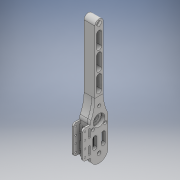
# Autodesk Inventor part: Arm - forearm v2
Saved by Autodesk Inventor 2017 (Build 210142000, 142)
## iProperties
Created: 2016-08-12
Part Number: Arm - forearm v2
Material: Generic
Document SubType Name: Modeling
Designer: Ali
Density: 1 g/cm^3
Appearance: Default
Author: Ali
Autodesk Inventor part; units mm, degrees
ref_plane "YZ Plane" through (0, 0, 0) normal (1, 0, 0) x (0, 1, 0)
ref_plane "XZ Plane" through (0, 0, 0) normal (0, 1, 0) x (-1, 0, 0)
ref_plane "XY Plane" through (0, 0, 0) normal (0, 0, 1) x (1, 0, 0)
sketch "Sketch1" plane through (0, 0, 0) normal (1, 0, 0) x (0, 1, 0)
  line L0 (0, 160) -> (0, -54.4) construction
  line L1 (-8, 160) -> (-8, 40)
  arc A0 (8, 160) -> (-8, 160) centre (0, 160) ccw
  circle A1 centre (0, 0) radius 11
  circle A2 centre (0, 0) radius 17 construction
  arc A3 (8, 40) -> (15.3617, 7.2814) centre (84.3889, 40) ccw
  arc A4 (-15.3617, 7.2814) -> (-8, 40) centre (-84.3889, 40) ccw
  line L2 (0, 0) -> (0, -54.4) construction
  line L3 (-17, 0) -> (-17, -54.4)
  line L4 (17, -54.4) -> (17, 0)
  arc A5 (-17, -54.4) -> (17, -54.4) centre (0, -54.4) ccw
  arc A6 (17, 0) -> (15.3617, 7.2814) centre (0, 0) ccw
  arc A7 (-15.3617, 7.2814) -> (-17, 0) centre (0, 0) ccw
  line L5 (8, 40) -> (8, 160)
  line L6 (-8, 40) -> (8, 40) construction
  point P0 (0, 52.8)
  point P1 (0, -27.2)
  dimension "d0" = 160
  dimension "d1" = 54.4
  dimension "d2" = 22
  dimension "d3" = 6
  dimension "d5" = 34
  dimension "d6" = 16
  dimension "d7" = 40
  constraints: 18 end point, 14 point on circle, 8 centre point, 8 tangent, 3 coincident, 3 vertical, 2 midpoint, 2 parallel, 1 collinear, 1 horizontal, 1 point on line
  measures "d0" distance of point (0, 0) L0.start
  measures "d1" distance of L0.end point (0, 0)
  measures "d2" diameter of A1
  measures "d3" radial gap between concentric circles of A1 A2
  measures "d5" distance between parallel lines of L4 L3
  measures "d6" distance between parallel lines of L5 L1
  measures "d7" distance from line of point (0, 0) L6
extrude "Extrusion1" add sketch "Sketch1" along normal mid plane 20.6
hole "Hole1" at (10.3, 0, 160) direction (-1, 0, 0) diameter 4.3 end through all
sketch "Sketch2" plane through (0, 0, 0) normal (1, 0, 0) x (0, 1, 0)
  circle A0 centre (0, 0) radius 11 projected
extrude "Extrusion2" add sketch "Sketch2" along normal mid plane 6.6
hole "Hole3" at (3.3, 0, 0) direction (-1, 0, 0) diameter 12 end through all
sketch "Sketch3" plane through (10.3, 0, 0) normal (1, 0, 0) x (0, 0, -1)
  line L0 (54.4, 17) -> (0, 17) projected
  arc A0 (54.4, -17) -> (54.4, 17) centre (54.4, 0) ccw projected
  line L1 (0, -17) -> (54.4, -17) projected
  circle A1 centre (0, 0) radius 11 projected
  arc A2 (-7.2814, -15.3617) -> (-40, -8) centre (-40, -84.3889) ccw projected
  arc A3 (-40, 8) -> (-7.2814, 15.3617) centre (-40, 84.3889) ccw projected
  line L2 (-40, 8) -> (-40, -8)
  arc A4 (0, 17) -> (-7.2814, 15.3617) centre (0, 0) ccw projected
  arc A5 (-7.2814, -15.3617) -> (0, -17) centre (0, 0) ccw projected
  constraints: 4 end point, 2 point on circle
extrude "Extrusion3" add sketch "Sketch3" against normal blind 6 separate body
extrude "Extrusion4" cut sketch "Sketch3" against normal blind 6 bodies 1
hole "Hole4" at (10.3, 0, -54.4) direction (-1, 0, 0) diameter 4.3 end through all counterbore diameter 7.1 counterbore depth 4.1 bodies 2 1
sketch "Sketch4" plane through (4.3, 0, 0) normal (1, 0, 0) x (0, 0, -1)
  circle A0 centre (0, 0) radius 11 projected
  line L0 (0, 17) -> (54.4, 17) projected
  arc A1 (54.4, -17) -> (54.4, 17) centre (54.4, 0) ccw projected
  line L1 (54.4, -17) -> (0, -17) projected
  arc A2 (12.3288, -17) -> (12.3288, 17) centre (0, 0) ccw
  dimension "d53" = 10
  constraints: 2 point on circle, 2 point on line, 1 centre point, 1 coincident
  measures "d53" radial gap between concentric circles of A2 A0
extrude "Extrusion5" cut sketch "Sketch4" against normal blind 8.6 contours L0 A1 L1 A2 bodies 1
sketch "Sketch5" plane through (10.3, 0, 0) normal (1, 0, 0) x (0, 0, -1)
  point P0 (0, 0)
  point P1 (-24, 0)
  point P2 (10, 12)
  point P3 (10, -12)
  dimension "d56" = 12
  dimension "d57" = 12
  dimension "d58" = 24
  dimension "d59" = 10
  dimension "d60" = 10
  measures "d56" vertical distance of point (10, 12) point (0, 0)
  measures "d57" vertical distance of point (10, -12) point (0, 0)
  measures "d58" distance of point (0, 0) point (-24, 0)
  measures "d59" horizontal distance of point (10, 12) point (0, 0)
  measures "d60" horizontal distance of point (10, -12) point (0, 0)
hole "Hole5" at (10.3, 0, 0) at (10.3, 0, 24) at (10.3, 12, -10) at (10.3, -12, -10) direction (-1, 0, 0) diameter 3.2 end through all counterbore diameter 6 counterbore depth 3.2 bodies 2 1
sketch "Sketch6" plane through (-10.3, 0, 0) normal (-1, 0, 0) x (0, 0, 1)
  circle A0 centre (-10, 12) radius 1.6 projected
  circle A1 centre (-10, 12) radius 3 projected
  line L0 (-7, 10.2679) -> (-10, 8.5359)
  line L1 (-10, 8.5359) -> (-13, 10.2679)
  line L2 (-13, 10.2679) -> (-13, 13.7321)
  line L3 (-13, 13.7321) -> (-10, 15.4641)
  line L4 (-10, 15.4641) -> (-7, 13.7321)
  line L5 (-7, 13.7321) -> (-7, 10.2679)
  circle A2 centre (-10, -12) radius 1.6 projected
  circle A3 centre (-10, -12) radius 3 projected
  line L6 (-7, -13.7321) -> (-10, -15.4641)
  line L7 (-10, -15.4641) -> (-13, -13.7321)
  line L8 (-13, -13.7321) -> (-13, -10.2679)
  line L9 (-13, -10.2679) -> (-10, -8.5359)
  line L10 (-10, -8.5359) -> (-7, -10.2679)
  line L11 (-7, -10.2679) -> (-7, -13.7321)
  circle A4 centre (24, 0) radius 3 projected
  line L12 (27, -1.7321) -> (24, -3.4641)
  line L13 (24, -3.4641) -> (21, -1.7321)
  line L14 (21, -1.7321) -> (21, 1.7321)
  line L15 (21, 1.7321) -> (24, 3.4641)
  line L16 (24, 3.4641) -> (27, 1.7321)
  line L17 (27, 1.7321) -> (27, -1.7321)
  point P0 (0, 0)
  point P1 (-7, 12)
  point P2 (-7, -12)
  point P3 (27, 0)
  constraints: 36 end point, 3 coincident, 3 horizontal alignment, 3 midpoint, 1 point on line, 42 other
extrude "Extrusion6" cut sketch "Sketch6" against normal blind 5 bodies 1
sketch "Sketch7" plane through (-10.3, 0, 0) normal (-1, 0, 0) x (0, 0, 1)
  circle A0 centre (-54.4, 0) radius 2.15 projected
  circle A1 centre (-54.4, 0) radius 3.55 projected
  line L0 (-50.85, -2.0496) -> (-54.4, -4.0992)
  line L1 (-54.4, -4.0992) -> (-57.95, -2.0496)
  line L2 (-57.95, -2.0496) -> (-57.95, 2.0496)
  line L3 (-57.95, 2.0496) -> (-54.4, 4.0992)
  line L4 (-54.4, 4.0992) -> (-50.85, 2.0496)
  line L5 (-50.85, 2.0496) -> (-50.85, -2.0496)
  point P0 (0, 0)
  point P1 (-50.85, 0)
  constraints: 12 end point, 1 coincident, 1 horizontal alignment, 1 midpoint, 14 other
extrude "Extrusion7" cut sketch "Sketch7" against normal blind 4 bodies 1
sketch "Sketch8" plane through (10.3, 0, 0) normal (1, 0, 0) x (0, 0, -1)
  line L0 (-160, -5.6569) -> (-154.3431, 0)
  line L1 (-154.3431, 0) -> (-160, 5.6569)
  line L2 (-160, 5.6569) -> (-165.6569, 0)
  line L3 (-165.6569, 0) -> (-160, -5.6569)
  line L4 (-154.3431, 0) -> (-165.6569, 0) construction
  circle A0 centre (-160, 0) radius 2.15 projected
  point P0 (0, 0)
  point P1 (-160, 0)
  dimension "d74" = 8
  constraints: 10 end point, 2 parallel, 2 perpendicular, 1 coincident, 1 horizontal, 1 midpoint
  measures "d74" distance between parallel lines of L2 L0
extrude "Extrusion8" cut sketch "Sketch8" against normal blind 4 bodies 1
mirror "Mirror1" about plane through (0, 0, 0) normal (1, 0, 0) of "Extrusion8" bodies 1
sketch "Sketch9" plane through (-10.3, 0, 0) normal (-1, 0, 0) x (0, 0, 1)
  line L0 (-54.4, -17) -> (0, -17) projected
  line L1 (0, 17) -> (-54.4, 17) projected
  line L2 (-25.7926, -8) -> (-41.7926, -8) construction
  line L3 (-25.7926, -4) -> (-41.7926, -4)
  line L4 (-41.7926, -12) -> (-25.7926, -12)
  arc A0 (-25.7926, -12) -> (-25.7926, -4) centre (-25.7926, -8) ccw
  arc A1 (-41.7926, -4) -> (-41.7926, -12) centre (-41.7926, -8) ccw
  line L5 (0, 0) -> (-49.4769, 0)
  line L6 (-25.7926, 8) -> (-41.7926, 8) construction
  line L7 (-25.7926, 4) -> (-41.7926, 4)
  line L8 (-41.7926, 12) -> (-25.7926, 12)
  arc A2 (-25.7926, 4) -> (-25.7926, 12) centre (-25.7926, 8) ccw
  arc A3 (-41.7926, 12) -> (-41.7926, 4) centre (-41.7926, 8) ccw
  point P0 (-33.7926, -8)
  point P1 (-33.7926, 8)
  dimension "d77" = 8
  dimension "d78" = 16
  dimension "d79" = 8
  constraints: 18 end point, 8 point on circle, 7 symmetric about line, 4 centre point, 4 tangent, 2 horizontal, 1 midpoint, 1 parallel, 2 other
  measures "d77" diameter of A1
  measures "d78" distance of L2.start L2.end
  measures "d79" distance between parallel lines of L3 L7
extrude "Extrusion9" cut sketch "Sketch9" against normal through all bodies 1 2
sketch "Sketch10" plane through (-10.3, 0, 0) normal (-1, 0, 0) x (0, 0, 1)
  line L0 (-54.4, -17) -> (0, -17) projected
  line L1 (0, -17) -> (-54.4, -17)
  line L2 (-54.4, -17) -> (-54.4, -31)
  line L3 (-54.4, -31) -> (0, -31)
  line L4 (0, -31) -> (0, -17)
  line L5 (-6, -18.5) -> (-20.1333, -18.5) construction
  line L6 (-6, -17) -> (-20.1333, -17)
  line L7 (-20.1333, -20) -> (-6, -20)
  arc A0 (-6, -20) -> (-6, -17) centre (-6, -18.5) ccw
  arc A1 (-20.1333, -17) -> (-20.1333, -20) centre (-20.1333, -18.5) ccw
  line L8 (-34.2667, -18.5) -> (-48.4, -18.5) construction
  line L9 (-34.2667, -17) -> (-48.4, -17)
  line L10 (-48.4, -20) -> (-34.2667, -20)
  arc A2 (-34.2667, -20) -> (-34.2667, -17) centre (-34.2667, -18.5) ccw
  arc A3 (-48.4, -17) -> (-48.4, -20) centre (-48.4, -18.5) ccw
  point P0 (0, 0)
  point P1 (-13.0667, -18.5)
  point P2 (-41.3333, -18.5)
  dimension "d82" = 14
  dimension "d83" = 3
  dimension "d84" = 1.5
  dimension "d85" = 6
  dimension "d86" = 6
  dimension "d88" = 42.4
  dimension "d89" = 14.1333
  dimension "d90" = 14.1333
  constraints: 24 end point, 8 point on circle, 8 tangent, 4 centre point, 4 parallel, 3 point on line, 2 horizontal, 2 midpoint, 1 collinear, 1 perpendicular
  measures "d82" distance between parallel lines of L3 L0
  measures "d83" diameter of A1
  measures "d84" radius of A2
  measures "d85" distance from line of L4 L5.start
  measures "d86" distance from line of L2 L8.end
  measures "d88" distance of L8.end L5.start
  measures "d89" distance of L5.start L5.end
  measures "d90" distance of L8.start L8.end
extrude "Extrusion10" add sketch "Sketch10" against normal blind 3 contours L0 A3 L10 A2 A1 L7 A0 L4 L3 L2 bodies 1
sketch "Sketch11" plane through (-10.3, 0, 0) normal (-1, 0, 0) x (0, 0, 1)
  line L0 (0, -27) -> (-54.4, -27)
  line L1 (-54.4, -31) -> (-54.4, -17) projected
  line L2 (-54.4, -31) -> (0, -31) projected
  line L3 (0, -31) -> (0, -17) projected
  point P0 (0, 0)
  point P1 (-6, -27)
  point P2 (-48.4, -27)
  point P3 (-20.1333, -27)
  point P4 (-34.2667, -27)
  dimension "d93" = 4
  dimension "d94" = 6
  dimension "d95" = 6
  dimension "d96" = 42.4
  dimension "d97" = 14.1333
  dimension "d98" = 14.1333
  constraints: 5 point on line, 2 end point, 1 horizontal
  measures "d93" distance between parallel lines of L2 L0
  measures "d94" distance from line of L3 point (-6, -27)
  measures "d95" distance from line of L1 point (-48.4, -27)
  measures "d96" distance of point (-48.4, -27) point (-6, -27)
  measures "d97" distance of point (-6, -27) point (-20.133, -27)
  measures "d98" distance of point (-20.133, -27) point (-34.267, -27)
hole "Hole6" at (-10.3, -27, -6) at (-10.3, -27, -48.4) at (-10.3, -27, -20.1333) at (-10.3, -27, -34.2667) direction (1, 0, 0) diameter 3.2 end through all bodies 1
mirror "Mirror2" about plane through (0, 0, 0) normal (1, 0, 0) of "Extrusion10", "Hole6" bodies 2
fillet "Fillet2" radius 5 4 edges at (-8.8, -31, -54.4) (-8.8, -31, 0) (8.8, -31, -54.4) (8.8, -31, 0)
fillet "Fillet3" radius 11 2 edges at (0, -17, -12.3288) (0, 17, -12.3288)
sketch "Sketch12" plane through (-10.3, 0, 0) normal (-1, 0, 0) x (0, 0, 1)
  line L0 (40, -8) -> (160, -8) projected
  arc A0 (160, -8) -> (160, 8) centre (160, 0) ccw projected
  line L1 (160, 8) -> (40, 8) projected
  line L2 (40, -5) -> (160, -5)
  arc A1 (160, -5) -> (160, 5) centre (160, 0) ccw
  line L3 (160, 5) -> (40, 5)
  line L4 (144, 0) -> (121, 0) construction
  line L5 (144, 5) -> (121, 5)
  line L6 (121, -5) -> (144, -5)
  arc A2 (144, -5) -> (144, 5) centre (144, 0) ccw
  arc A3 (121, 5) -> (121, -5) centre (121, 0) ccw
  line L7 (108, 0) -> (85, 0) construction
  line L8 (108, 5) -> (85, 5)
  line L9 (85, -5) -> (108, -5)
  arc A4 (108, -5) -> (108, 5) centre (108, 0) ccw
  arc A5 (85, 5) -> (85, -5) centre (85, 0) ccw
  line L10 (72, 0) -> (49, 0) construction
  line L11 (72, 5) -> (49, 5)
  line L12 (49, -5) -> (72, -5)
  arc A6 (72, -5) -> (72, 5) centre (72, 0) ccw
  arc A7 (49, 5) -> (49, -5) centre (49, 0) ccw
  point P0 (0, 0)
  point P1 (132.5, 0)
  point P2 (96.5, 0)
  point P3 (60.5, 0)
  dimension "d109" = 3
  dimension "d110" = 13
  dimension "d111" = 13
  dimension "d112" = 23
  dimension "d113" = 23
  dimension "d114" = 23
  dimension "d115" = 16
  constraints: 28 end point, 14 point on circle, 12 tangent, 7 centre point, 4 collinear, 4 point on line, 3 midpoint, 3 parallel, 1 horizontal, 2 other
  measures "d109" distance between parallel lines of L0 L2
  measures "d110" distance of L7.start L4.end
  measures "d111" distance of L10.start L7.end
  measures "d112" distance of L4.start L4.end
  measures "d113" distance of L7.start L7.end
  measures "d114" distance of L10.start L10.end
  measures "d115" distance of A0.centre L4.start
extrude "Extrusion11" cut sketch "Sketch12" against normal through all contours A7 L3 A6 L2 | A5 L3 A4 L2 | A3 L3 A2 L2 bodies 1
equation "\"d59\" = d60"
equation "\"d86\" = d85"
equation "\"d89\" = 0.333333 * d88"
equation "\"d90\" = d89"
equation "\"d97\" = 0.333333 * d96"
equation "\"d98\" = d97"
equation "\"d111\" = d110"
equation "\"d113\" = d112"
equation "\"d114\" = d113"
